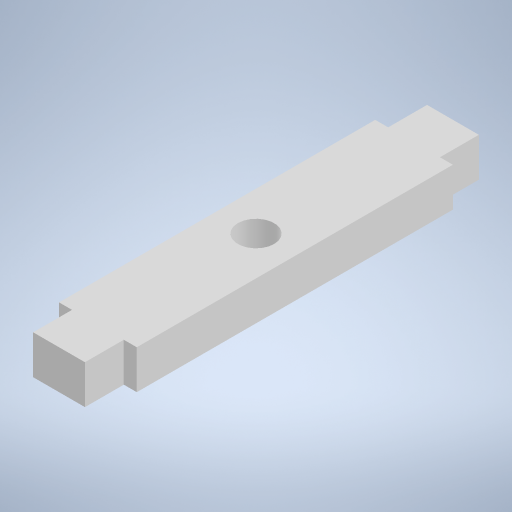
# Autodesk Inventor part: 螺絲
Saved by Autodesk Inventor 2023 (Build 270158000, 158)
## iProperties
Created: 2024-03-31
Part Number: 螺絲
Material: 一般
Document SubType Name: Modeling
Designer: USER
Density: 1 g/cm^3
Appearance: 預設
Author: USER
Autodesk Inventor part; units mm, degrees
ref_plane "YZ Plane" through (0, 0, 0) normal (1, 0, 0) x (0, 1, 0)
ref_plane "XZ Plane" through (0, 0, 0) normal (0, 1, 0) x (-1, 0, 0)
ref_plane "XY Plane" through (0, 0, 0) normal (0, 0, 1) x (1, 0, 0)
sketch "草圖1" plane through (0, 0, 0) normal (0, 1, 0) x (-1, 0, 0)
  line L0 (0, 0) -> (6, 0)
  line L1 (6, 0) -> (6, -24.4)
  line L2 (6, -24.4) -> (0, -24.4)
  line L3 (0, -24.4) -> (0, 0)
  line L4 (1, 0) -> (5, 0)
  line L5 (5, 0) -> (5, 3)
  line L6 (5, 3) -> (1, 3)
  line L7 (1, 3) -> (1, 0)
  line L8 (5, -24.4) -> (1, -24.4)
  line L9 (1, -24.4) -> (1, -27.4)
  line L10 (1, -27.4) -> (5, -27.4)
  line L11 (5, -27.4) -> (5, -24.4)
  line L12 (3, 0) -> (3, -24.4)
  line L13 (6, -12.2) -> (0, -12.2)
  circle A0 centre (3, -12.2) radius 1.4
  dimension "d0" = 24.4
  dimension "d1" = 6
  dimension "d2" = 4
  dimension "d3" = 3
  dimension "d4" = 3
  dimension "d5" = 4
  dimension "d6" = 2.8
  constraints: 28 end point, 7 midpoint, 6 parallel, 4 perpendicular, 3 horizontal, 1 centre point
  measures "d0" distance of L2.end L0.start
  measures "d1" distance of L0.start L0.end
  measures "d2" distance of L5.end L6.end
  measures "d3" distance of L4.end L5.end
  measures "d4" distance of L8.end L9.end
  measures "d5" distance of L9.end L10.end
  measures "d6" diameter of A0
extrude "擠出1" add sketch "草圖1" along normal blind 3 contours L0 L12 A0 L13 L3 | L7 L6 L5 L0 | L13 A0 L12 L2 L3 | L0 L1 L13 A0 L12 | L2 L11 L10 L9 | A0 L13 L1 L2 L12
